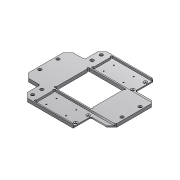
# Autodesk Inventor part: BC-10021
Saved by Autodesk Inventor 2016 (Build 200138000, 138)
## iProperties
Created: 2015-12-01
Part Number: BC-10021
Project: DIPOLO BC-3T- SIRIUS
Cost Center: 1504002005
Material: Alumínio 7075
Document SubType Name: Modeling
Designer: reinaldo.basilio
Density: 2.81 g/cm^3
Appearance: Aluminum - Polished
Mass: 835.488 g
Surface Area: 1001.25 cm^2
Volume: 297.327 cm^3
Description: Tampa de proteção dos blocos e guia dos compesadores de gradiente.
RuleStatus: InUse
AfterMaterialChange0: file://_iMaterial
AfterAnyiPropertyChange0: file://_iMaterial
AfterDocNew0: file://_Naming_par
AfterDocNew1: file://_NameStart
AfterDocNew2: file://_NameStart1
AfterDocNew3: file://_Materiais
DocNumber: XXXXX-XXX-XXXX-00-001.ipt
Folder: .
Title: DIPOLO BC-3T- SIRIUS
Author: reinaldo.basilio
Subject: BC-10021
Autodesk Inventor part; units mm, degrees
ref_plane "YZ Plane" through (0, 0, 0) normal (1, 0, 0) x (0, 1, 0)
ref_plane "XZ Plane" through (0, 0, 0) normal (0, 1, 0) x (-1, 0, 0)
ref_plane "XY Plane" through (0, 0, 0) normal (0, 0, 1) x (1, 0, 0)
sketch "Sketch5" plane through (0, 0, 0) normal (0, 0, 1) x (1, 0, 0)
  line L0 (-121.5, 134) -> (121.5, 134)
  line L1 (121.5, 134) -> (121.5, -134)
  line L2 (121.5, -134) -> (-121.5, -134)
  line L3 (-121.5, -134) -> (-121.5, 134)
  point P0 (0, 0)
  point P1 (0, 134)
  point P2 (121.5, 0)
  dimension "d8" = 243
  dimension "d43" = 268
  constraints: 8 end point, 2 midpoint, 2 parallel, 1 horizontal, 1 horizontal alignment, 1 perpendicular, 1 vertical alignment
  measures "d8" distance of L0.start L0.end
  measures "d43" distance between parallel lines of L0 L2
extrude "Extrusion5" add sketch "Sketch5" along normal blind 10
sketch "Sketch6" plane through (0, 0, 10) normal (0, 0, 1) x (1, 0, 0)
  line L0 (-52.5, 55) -> (52.5, 55)
  line L1 (52.5, 55) -> (52.5, -55)
  line L2 (52.5, -55) -> (-52.5, -55)
  line L3 (-52.5, -55) -> (-52.5, 55)
  arc A0 (46.5, -55) -> (52.5, -55) centre (49.5, -55) ccw
  arc A1 (-52.5, -55) -> (-46.5, -55) centre (-49.5, -55) ccw
  arc A2 (-46.5, 55) -> (-52.5, 55) centre (-49.5, 55) ccw
  arc A3 (52.5, 55) -> (46.5, 55) centre (49.5, 55) ccw
  point P0 (0, 0)
  point P1 (-52.5, 0)
  point P2 (0, -55)
  dimension "d12" = 105
  dimension "d13" = 110
  dimension "d108" = 6
  constraints: 8 end point, 8 point on circle, 8 point on line, 4 centre point, 4 tangent, 3 equal radius, 2 midpoint, 2 parallel, 1 horizontal, 1 horizontal alignment, 1 perpendicular, 1 vertical alignment
  measures "d12" distance of L0.start L0.end
  measures "d13" distance of L0.end L1.end
  measures "d108" diameter of A0
extrude "Extrusion6" cut sketch "Sketch6" against normal through all
sketch "Sketch7" plane through (0, 0, 10) normal (0, 0, 1) x (1, 0, 0)
  line L0 (121.5, 134) -> (-121.5, 134) projected
  line L1 (121.5, -134) -> (121.5, 134) projected
  line L2 (121.5, 70) -> (67.5, 70)
  line L3 (67.5, 70) -> (67.5, 134)
  line L4 (67.5, 134) -> (121.5, 134)
  line L5 (121.5, 134) -> (121.5, 70)
  line L6 (0, 0) -> (0, 14.6341) construction
  circle A0 centre (27.5, 125) radius 4.5
  circle A1 centre (-27.5, 125) radius 4.5
  line L7 (-121.5, 70) -> (-67.5, 70)
  line L8 (-67.5, 70) -> (-67.5, 134)
  line L9 (-67.5, 134) -> (-121.5, 134)
  line L10 (-121.5, 134) -> (-121.5, 70)
  line L11 (121.5, -134) -> (67.5, -134)
  line L12 (67.5, -134) -> (67.5, -84)
  line L13 (67.5, -84) -> (121.5, -84)
  line L14 (121.5, -84) -> (121.5, -134)
  circle A2 centre (27.5, -78) radius 4.5
  circle A3 centre (-27.5, -78) radius 4.5
  line L15 (-121.5, -134) -> (-67.5, -134)
  line L16 (-67.5, -134) -> (-67.5, -84)
  line L17 (-67.5, -84) -> (-121.5, -84)
  line L18 (-121.5, -84) -> (-121.5, -134)
  line L19 (-121.5, -134) -> (121.5, -134) projected
  point P0 (-121.5, -69)
  dimension "d23" = 64
  dimension "d63" = 67.5
  dimension "d88" = 50
  dimension "d89" = 54
  dimension "d90" = 54
  constraints: 34 end point, 5 collinear, 5 symmetric about line, 4 centre point, 4 parallel, 2 horizontal, 2 horizontal alignment, 2 perpendicular, 2 vertical
  measures "d23" distance of L4.end L2.start
  measures "d63" distance between parallel lines of L6 L3
  measures "d88" distance of L14.start L11.start
  measures "d89" distance of L12.end L14.start
  measures "d90" distance of L16.end L17.end
extrude "Extrusion7" cut sketch "Sketch7" against normal through all contours L1 L2 L3 L0 | L15 L18 L17 L16 | L1 L11 L12 L13 | L8 L7 L10 L0
sketch "Sketch8" plane through (0, 0, 10) normal (0, 0, 1) x (1, 0, 0)
  line L0 (0, 0) -> (0, 14.6341) construction
  circle A0 centre (27.5, -125) radius 4.5
  circle A1 centre (-27.5, -125) radius 4.5
  circle A2 centre (27.5, 125) radius 4.5
  circle A3 centre (-27.5, 125) radius 4.5
  circle A4 centre (76.5, -70) radius 4.5
  circle A5 centre (-76.5, -70) radius 4.5
  circle A6 centre (104.5, -70) radius 4.5
  circle A7 centre (-104.5, -70) radius 4.5
  dimension "d28" = 55
  dimension "d29" = 27.5
  dimension "d30" = 9
  dimension "d31" = 250
  dimension "d41" = 55
  dimension "d48" = 153
  dimension "d49" = 76.5
  dimension "d50" = 55
  dimension "d51" = 125
  dimension "d53" = 28
  dimension "d54" = 28
  constraints: 8 centre point, 7 equal radius, 5 horizontal alignment, 2 end point, 2 vertical alignment, 1 vertical
  measures "d28" distance of A1.centre A0.centre
  measures "d29" horizontal distance of L0.start A0.centre
  measures "d30" diameter of A0
  measures "d31" distance of A2.centre A0.centre
  measures "d41" distance of A3.centre A2.centre
  measures "d48" distance of A5.centre A4.centre
  measures "d49" horizontal distance of point (0, 0) A5.centre
  measures "d50" vertical distance of A4.centre A0.centre
  measures "d51" vertical distance of A1.centre point (0, 0)
  measures "d53" distance of A4.centre A6.centre
  measures "d54" distance of A7.centre A5.centre
hole "Hole1" at (27.5, -125, 10) at (-27.5, -125, 10) at (-27.5, 125, 10) at (27.5, 125, 10) at (104.5, -70, 10) at (76.5, -70, 10) at (-76.5, -70, 10) at (-104.5, -70, 10) direction (0, 0, -1) diameter 5.5 end through all counterbore diameter 10 counterbore depth 5.5 clearance for "Socket Head Cap Screw DIN EN ISO 4762" size "M5" standard "DIN"
chamfer "Chamfer1" distance 15 angle 45 4 edges at (-67.5, 134, 5) (67.5, 134, 5) (67.5, -134, 5) (-67.5, -134, 5)
fillet "Fillet2" radius 4 4 edges at (67.5, 70, 5) (-67.5, 70, 5) (67.5, -84, 5) (-67.5, -84, 5)
sketch "Sketch10" plane through (0, 0, 10) normal (0, 0, 1) x (1, 0, 0)
  line L0 (121.5, -84) -> (121.5, 70) projected
  line L1 (118.5, -50) -> (56, -50)
  line L2 (56, -50) -> (56, 134)
  line L3 (56, 134) -> (118.5, 134)
  line L4 (118.5, 134) -> (118.5, -50)
  line L5 (0, 0) -> (0, -20.3736) construction
  line L6 (-118.5, -50) -> (-56, -50)
  line L7 (-56, -50) -> (-56, 134)
  line L8 (-56, 134) -> (-118.5, 134)
  line L9 (-118.5, 134) -> (-118.5, -50)
  line L10 (52.5, 134) -> (-52.5, 134) projected
  arc A0 (112.5, -50) -> (118.5, -50) centre (115.5, -50) ccw
  arc A1 (56, -50) -> (62, -50) centre (59, -50) ccw
  circle A2 centre (-115.5, -50) radius 3
  circle A3 centre (-59, -50) radius 3
  point P0 (-112.5, -50)
  dimension "d57" = 62.5
  dimension "d59" = 56
  dimension "d60" = 3
  dimension "d101" = 50
  dimension "d107" = 6
  constraints: 18 end point, 7 symmetric about line, 6 point on circle, 4 point on line, 3 centre point, 2 parallel, 2 tangent, 1 collinear, 1 equal radius, 1 horizontal, 1 horizontal alignment, 1 perpendicular, 1 vertical, 4 other
  measures "d57" distance of L2.end L3.end
  measures "d59" distance from line of L5.start L2
  measures "d60" distance between parallel lines of L4 L0
  measures "d101" distance from line of L5.start L1
  measures "d107" diameter of A0
extrude "Extrusion8" cut sketch "Sketch10" against normal blind 6.3
sketch "Sketch11" plane through (0, 0, 3.7) normal (0, 0, 1) x (1, 0, 0)
  line L0 (56, -50) -> (56, 130.5) projected
  line L1 (118.5, -50) -> (56, -50) projected
  circle A0 centre (102.75, -30) radius 2
  circle A1 centre (71.75, -30) radius 2
  circle A2 centre (102.75, 30) radius 2
  circle A3 centre (71.75, 30) radius 2
  line L2 (0, 0) -> (0, -13.697) construction
  circle A4 centre (-102.75, -30) radius 2
  circle A5 centre (-71.75, -30) radius 2
  circle A6 centre (-102.75, 30) radius 2
  circle A7 centre (-71.75, 30) radius 2
  point P0 (57.5, 50)
  point P1 (56, 130.5)
  dimension "d65" = 60
  dimension "d66" = 20
  dimension "d67" = 31
  dimension "d68" = 15.75
  dimension "d69" = 4
  constraints: 8 centre point, 4 symmetric about line, 3 equal radius, 2 end point, 2 horizontal alignment, 2 vertical alignment, 1 vertical, 5 other
  measures "d65" distance of A2.centre A0.centre
  measures "d66" distance from line of L1 A0.centre
  measures "d67" distance of A1.centre A0.centre
  measures "d69" diameter of A0
hole "Hole2" at (102.75, -30, 3.7) at (71.75, -30, 3.7) at (71.75, 30, 3.7) at (102.75, 30, 3.7) at (-71.75, 30, 3.7) at (-102.75, 30, 3.7) at (-102.75, -30, 3.7) at (-71.75, -30, 3.7) direction (0, 0, -1) diameter 3.242 end through all thread size "M4x0.7" class "6H" standard "ISO Metric profile"
sketch "Sketch12" plane through (0, 0, 3.7) normal (0, 0, 1) x (1, 0, 0)
  line L0 (121.5, 70) -> (71.5, 70)
  circle A0 centre (106, 62.5) radius 3
  line L1 (0, 0) -> (0, 4.9934) construction
  circle A1 centre (-106, 62.5) radius 3
  circle A2 centre (67.5, 62.5) radius 3
  line L2 (-52.5, -55) -> (-52.5, 55) projected
  line L3 (46.5, -55) -> (-46.5, -55) projected
  circle A3 centre (-67.5, 62.5) radius 3
  point P0 (121.5, -134)
  point P1 (-52.5, 0)
  point P2 (0, -55)
  dimension "d78" = 7.5
  dimension "d80" = 6
  dimension "d98" = 106
  dimension "d99" = 106
  dimension "d105" = 6
  dimension "d106" = 38.5
  constraints: 4 centre point, 4 end point, 2 horizontal alignment, 2 midpoint, 2 symmetric about line, 1 vertical, 1 vertical alignment, 3 other
  measures "d78" distance from line of L0 A0.centre
  measures "d80" diameter of A0
  measures "d98" distance from line of L1 A0.centre
  measures "d99" distance from line of A1.centre L1
  measures "d105" diameter of A2
  measures "d106" distance of A2.centre A0.centre
hole "Hole3" at (106, 62.5, 3.7) at (-106, 62.5, 3.7) at (67.5, 62.5, 3.7) at (-67.5, 62.5, 3.7) direction (0, 0, -1) diameter 5.5 end through all countersink diameter 11 countersink angle 90 clearance for "Countersunk Flat Head Screw DIN EN ISO 2009" size "M5" standard "DIN"
chamfer "Chamfer5" distance 15 angle 45 2 edges at (121.5, -84, 5) (-121.5, -84, 5)
chamfer "Chamfer6" distance 3 angle 45 2 edges at (120, 70, 10) (-120, 70, 10)
equation "\"d90\" = d89"
equation "\"d29\" = 0.5 * d28"
equation "\"d49\" = 0.5 * d48"
equation "\"d51\" = 0.5 * d31"
body "Solid5"
